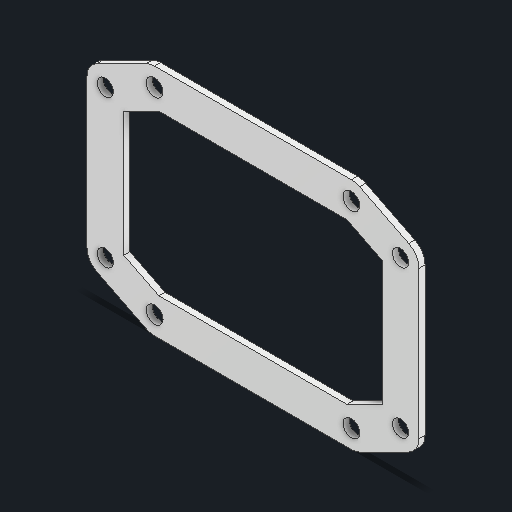
# Autodesk Inventor part: Brain Mount
Saved by Autodesk Inventor 2025.1 (Build 291241000, 241)
## iProperties
Created: 2024-11-19
Part Number: Brain Mount
Material: Acetal Resin, White
Document SubType Name: Modeling
Designer: avere
Density: 1.425 g/cm^3
Appearance: Smooth - White
Author: avere
Autodesk Inventor part; units mm, degrees
ref_plane "YZ Plane" through (0, 0, 0) normal (1, 0, 0) x (0, 1, 0)
ref_plane "XZ Plane" through (0, 0, 0) normal (0, 1, 0) x (-1, 0, 0)
ref_plane "XY Plane" through (0, 0, 0) normal (0, 0, 1) x (1, 0, 0)
sketch "Sketch1" plane through (0, 0, 0) normal (0, 0, 1) x (1, 0, 0)
  circle A0 centre (-38.5364, -16.421) radius 2.0955
  circle A1 centre (-38.5364, 21.679) radius 2.0955
  circle A2 centre (37.6731, -16.4179) radius 2.0955
  circle A3 centre (37.6731, 21.6821) radius 2.0955
  circle A4 centre (-25.8269, -22.7679) radius 2.1844
  circle A5 centre (24.9731, -22.7679) radius 2.1844
  circle A6 centre (24.9731, 28.0321) radius 2.1844
  circle A7 centre (-25.8269, 28.0321) radius 2.1844
  arc A8 (-25.8269, 32.7946) -> (-27.9563, 32.2921) centre (-25.8269, 28.0321) ccw
  arc A9 (27.103, 32.2919) -> (24.9731, 32.7946) centre (24.9731, 28.0321) ccw
  arc A10 (42.4356, 21.6821) -> (39.803, 25.9419) centre (37.6731, 21.6821) ccw
  arc A11 (39.803, -20.6776) -> (42.4356, -16.4179) centre (37.6731, -16.4179) ccw
  arc A12 (24.9731, -27.5304) -> (27.103, -27.0276) centre (24.9731, -22.7679) ccw
  arc A13 (-27.9546, -27.0286) -> (-25.8269, -27.5304) centre (-25.8269, -22.7679) ccw
  arc A14 (-43.2989, -16.421) -> (-40.6641, -20.6818) centre (-38.5364, -16.421) ccw
  arc A15 (-40.6658, 25.9389) -> (-43.2989, 21.679) centre (-38.5364, 21.679) ccw
  line L0 (-43.2989, 21.679) -> (-43.2989, -16.421)
  line L1 (-40.6641, -20.6818) -> (-27.9546, -27.0286)
  line L2 (-40.6658, 25.9389) -> (-27.9563, 32.2921)
  line L3 (-25.8269, 32.7946) -> (24.9731, 32.7946)
  line L4 (27.103, 32.2919) -> (39.803, 25.9419)
  line L5 (39.803, -20.6776) -> (27.103, -27.0276)
  line L6 (42.4356, -16.4179) -> (42.4356, 21.6821)
  line L7 (-25.8269, -27.5304) -> (24.9731, -27.5304)
  line L8 (-24.7028, 23.2696) -> (-33.7739, 18.7353)
  line L9 (-33.7739, 18.7353) -> (-33.7739, -13.476)
  line L10 (-33.7739, -13.476) -> (-24.7039, -18.0054)
  line L11 (-24.7039, -18.0054) -> (23.8489, -18.0054)
  line L12 (23.8489, -18.0054) -> (32.9106, -13.4745)
  line L13 (32.9106, -13.4745) -> (32.9106, 18.7388)
  line L14 (32.9106, 18.7388) -> (23.8489, 23.2696)
  line L15 (23.8489, 23.2696) -> (-24.7028, 23.2696)
  point P0 (0, 0)
  dimension "d9" = 9.525
  dimension "d10" = 9.525
  dimension "d11" = 9.525
  dimension "d12" = 9.525
  dimension "d13" = 9.525
  dimension "d14" = 9.525
  dimension "d15" = 9.525
  dimension "d16" = 9.525
  dimension "d17" = 9.525
  constraints: 37 end point, 16 centre point, 16 point on circle, 11 tangent, 8 coincident, 2 perpendicular, 22 other
  measures "d9" diameter of A8
  measures "d10" diameter of A9
  measures "d11" diameter of A10
  measures "d12" diameter of A11
  measures "d13" diameter of A12
  measures "d14" diameter of A13
  measures "d15" diameter of A14
  measures "d16" diameter of A15
  measures "d17" distance between parallel lines of L2 L8
extrude "Extrusion1" add sketch "Sketch1" along normal blind 1.5875
body "Solid1"
